Autodesk Fusion 360 part; units mm, degrees
(part 2 of 2)
sketch "Sketch5" plane through (0, 0, 0) normal (0, 0, -1) x (1, 0, 0)
  line L0 (-3.9005, -90.0072) -> (0, -96.4395)
  line L1 (0, -96.4395) -> (3.9005, -90.0072)
  arc A0 (-3.9005, -90.0072) -> (3.9005, -90.0072) centre (0, -96.4395) ccw
  line L2 (-4.2635, 5.5365) -> (-12.4173, 13.98)
  line L3 (-12.4173, 13.98) -> (-12.6168, 25.4085)
  line L4 (-12.6168, 25.4085) -> (-12.6168, 30.4597)
  line L5 (-12.6168, 30.4597) -> (-9.0451, 26.888)
  line L6 (-9.0451, 26.888) -> (-1.105, 18.6658)
  line L7 (-1.105, 18.6658) -> (-0.9001, 6.9296)
  line L8 (-0.9001, 6.9296) -> (-0.9137, 6.1554)
  line L9 (-0.9137, 6.1554) -> (-1.6405, 5.2892)
  line L10 (-1.6405, 5.2892) -> (-2.0296, 4.9)
  line L11 (-2.0296, 4.9) -> (-2.58, 4.9)
  line L12 (-2.58, 4.9) -> (-3.7064, 4.9985)
  line L13 (-3.7064, 4.9985) -> (-4.2635, 5.5365)
  line L14 (-28.1497, 7.7612) -> (-21.2885, 0.9)
  line L15 (-21.2885, 0.9) -> (-31.2992, 0.9)
  line L16 (-31.2992, 0.9) -> (-41.9773, 11.2116)
  line L17 (-41.9773, 11.2116) -> (-40.4166, 12.6168)
  line L18 (-40.4166, 12.6168) -> (-33.1778, 12.6168)
  line L19 (-33.1778, 12.6168) -> (-28.1497, 7.7612)
  line L20 (-21.2885, -0.9) -> (-28.1497, -7.7612)
  line L21 (-28.1497, -7.7612) -> (-33.1778, -12.6168)
  line L22 (-33.1778, -12.6168) -> (-40.4166, -12.6168)
  line L23 (-40.4166, -12.6168) -> (-41.9773, -11.2116)
  line L24 (-41.9773, -11.2116) -> (-31.2992, -0.9)
  line L25 (-31.2992, -0.9) -> (-21.2885, -0.9)
  line L26 (-33.8904, -0.9) -> (-43.3182, -10.0043)
  line L27 (-43.3182, -10.0043) -> (-53.4295, -0.9)
  line L28 (-53.4295, -0.9) -> (-33.8904, -0.9)
  line L29 (-93.238, 0) -> (-86.2449, 4.2406)
  line L30 (-86.2449, 4.2406) -> (-75.7491, 0)
  line L31 (-75.7491, 0) -> (-86.2449, -4.2406)
  line L32 (-86.2449, -4.2406) -> (-93.238, 0)
  line L33 (-53.4295, 0.9) -> (-43.3182, 10.0043)
  line L34 (-43.3182, 10.0043) -> (-33.8904, 0.9)
  line L35 (-33.8904, 0.9) -> (-53.4295, 0.9)
  line L36 (-18.6658, 1.105) -> (-26.888, 9.0451)
  line L37 (-26.888, 9.0451) -> (-30.4597, 12.6168)
  line L38 (-30.4597, 12.6168) -> (-25.4085, 12.6168)
  line L39 (-25.4085, 12.6168) -> (-13.98, 12.4173)
  line L40 (-13.98, 12.4173) -> (-5.5365, 4.2635)
  line L41 (-5.5365, 4.2635) -> (-4.9985, 3.7064)
  line L42 (-4.9985, 3.7064) -> (-4.9, 2.58)
  line L43 (-4.9, 2.58) -> (-4.9, 2.0296)
  line L44 (-4.9, 2.0296) -> (-5.2892, 1.6405)
  line L45 (-5.2892, 1.6405) -> (-6.1554, 0.9137)
  line L46 (-6.1554, 0.9137) -> (-6.9296, 0.9001)
  line L47 (-6.9296, 0.9001) -> (-18.6658, 1.105)
  arc A1 (-6.182, -86.2449) -> (6.182, -86.2449) centre (0, -96.4395) ccw
  line L48 (6.182, -86.2449) -> (0.9, -73.1716)
  line L49 (0.9, -73.1716) -> (0.9, -66.6716)
  line L50 (0.9, -66.6716) -> (8.1008, -75.8883)
  arc A2 (8.1008, -75.8883) -> (9.5193, -74.7801) centre (8.8101, -75.3342) ccw
  line L51 (9.5193, -74.7801) -> (0.9, -63.7479)
  line L52 (0.9, -63.7479) -> (0.9, -56.6479)
  line L53 (0.9, -56.6479) -> (14.9397, -72.7987)
  arc A3 (14.9397, -72.7987) -> (16.2982, -71.6178) centre (15.6189, -72.2083) ccw
  line L54 (16.2982, -71.6178) -> (11.9485, -66.6141)
  line L55 (11.9485, -66.6141) -> (15.3003, -65.847)
  arc A4 (15.3003, -65.847) -> (14.8988, -64.0923) centre (15.0995, -64.9697) ccw
  line L56 (14.8988, -64.0923) -> (10.6097, -65.074)
  line L57 (10.6097, -65.074) -> (1.8798, -55.0314)
  line L58 (1.8798, -55.0314) -> (14.4168, -41.1076)
  line L59 (14.4168, -41.1076) -> (14.4168, -34.8053)
  line L60 (14.4168, -34.8053) -> (18.8732, -39.2617)
  line L61 (18.8732, -39.2617) -> (37.5839, -40.2423)
  line L62 (37.5839, -40.2423) -> (38.5121, -53.5164)
  line L63 (38.5121, -53.5164) -> (34.7851, -55.8551)
  arc A5 (34.7851, -55.8551) -> (35.7419, -57.3798) centre (35.2635, -56.6175) ccw
  line L64 (35.7419, -57.3798) -> (38.6544, -55.5521)
  line L65 (38.6544, -55.5521) -> (39.1169, -62.166)
  arc A6 (39.1169, -62.166) -> (40.9125, -62.0404) centre (40.0147, -62.1032) ccw
  line L66 (40.9125, -62.0404) -> (39.4198, -40.6925)
  line L67 (39.4198, -40.6925) -> (44.4402, -45.713)
  line L68 (44.4402, -45.713) -> (46.1464, -59.6086)
  arc A7 (46.1464, -59.6086) -> (47.933, -59.3893) centre (47.0397, -59.499) ccw
  line L69 (47.933, -59.3893) -> (46.5076, -47.7804)
  line L70 (46.5076, -47.7804) -> (51.1038, -52.3766)
  line L71 (51.1038, -52.3766) -> (56.6131, -65.3557)
  line L72 (56.6131, -65.3557) -> (68.193, -68.193)
  line L73 (68.193, -68.193) -> (65.3557, -56.6131)
  line L74 (65.3557, -56.6131) -> (52.3766, -51.1038)
  line L75 (52.3766, -51.1038) -> (47.7804, -46.5076)
  line L76 (47.7804, -46.5076) -> (59.3893, -47.933)
  arc A8 (59.3893, -47.933) -> (59.6086, -46.1464) centre (59.499, -47.0397) ccw
  line L77 (59.6086, -46.1464) -> (45.713, -44.4402)
  line L78 (45.713, -44.4402) -> (40.6925, -39.4198)
  line L79 (40.6925, -39.4198) -> (62.0404, -40.9125)
  arc A9 (62.0404, -40.9125) -> (62.166, -39.1169) centre (62.1032, -40.0147) ccw
  line L80 (62.166, -39.1169) -> (55.5521, -38.6544)
  line L81 (55.5521, -38.6544) -> (57.3798, -35.7419)
  arc A10 (57.3798, -35.7419) -> (55.8551, -34.7851) centre (56.6175, -35.2635) ccw
  line L82 (55.8551, -34.7851) -> (53.5164, -38.5121)
  line L83 (53.5164, -38.5121) -> (40.2423, -37.5839)
  line L84 (40.2423, -37.5839) -> (39.2617, -18.8732)
  line L85 (39.2617, -18.8732) -> (34.8053, -14.4168)
  line L86 (34.8053, -14.4168) -> (41.1076, -14.4168)
  line L87 (41.1076, -14.4168) -> (55.0314, -1.8798)
  line L88 (55.0314, -1.8798) -> (65.074, -10.6097)
  line L89 (65.074, -10.6097) -> (64.0923, -14.8988)
  arc A11 (64.0923, -14.8988) -> (65.847, -15.3003) centre (64.9697, -15.0995) ccw
  line L90 (65.847, -15.3003) -> (66.6141, -11.9485)
  line L91 (66.6141, -11.9485) -> (71.6178, -16.2982)
  arc A12 (71.6178, -16.2982) -> (72.7987, -14.9397) centre (72.2083, -15.6189) ccw
  line L92 (72.7987, -14.9397) -> (56.6479, -0.9)
  line L93 (56.6479, -0.9) -> (63.7479, -0.9)
  line L94 (63.7479, -0.9) -> (74.7801, -9.5193)
  arc A13 (74.7801, -9.5193) -> (75.8883, -8.1008) centre (75.3342, -8.8101) ccw
  line L95 (75.8883, -8.1008) -> (66.6716, -0.9)
  line L96 (66.6716, -0.9) -> (73.1716, -0.9)
  line L97 (73.1716, -0.9) -> (86.2449, -6.182)
  line L98 (86.2449, -6.182) -> (96.4395, 0)
  line L99 (96.4395, 0) -> (86.2449, 6.182)
  line L100 (86.2449, 6.182) -> (73.1716, 0.9)
  line L101 (73.1716, 0.9) -> (66.6716, 0.9)
  line L102 (66.6716, 0.9) -> (75.8883, 8.1008)
  arc A14 (75.8883, 8.1008) -> (74.7801, 9.5193) centre (75.3342, 8.8101) ccw
  line L103 (74.7801, 9.5193) -> (63.7479, 0.9)
  line L104 (63.7479, 0.9) -> (56.6479, 0.9)
  line L105 (56.6479, 0.9) -> (72.7987, 14.9397)
  arc A15 (72.7987, 14.9397) -> (71.6178, 16.2982) centre (72.2083, 15.6189) ccw
  line L106 (71.6178, 16.2982) -> (66.6141, 11.9485)
  line L107 (66.6141, 11.9485) -> (65.847, 15.3003)
  arc A16 (65.847, 15.3003) -> (64.0923, 14.8988) centre (64.9697, 15.0995) ccw
  line L108 (64.0923, 14.8988) -> (65.074, 10.6097)
  line L109 (65.074, 10.6097) -> (55.0314, 1.8798)
  line L110 (55.0314, 1.8798) -> (41.1076, 14.4168)
  line L111 (41.1076, 14.4168) -> (34.8053, 14.4168)
  line L112 (34.8053, 14.4168) -> (39.2617, 18.8732)
  line L113 (39.2617, 18.8732) -> (40.2423, 37.5839)
  line L114 (40.2423, 37.5839) -> (53.5164, 38.5121)
  line L115 (53.5164, 38.5121) -> (55.8551, 34.7851)
  arc A17 (55.8551, 34.7851) -> (57.3798, 35.7419) centre (56.6175, 35.2635) ccw
  line L116 (57.3798, 35.7419) -> (55.5521, 38.6544)
  line L117 (55.5521, 38.6544) -> (62.166, 39.1169)
  arc A18 (62.166, 39.1169) -> (62.0404, 40.9125) centre (62.1032, 40.0147) ccw
  line L118 (62.0404, 40.9125) -> (40.6925, 39.4198)
  line L119 (40.6925, 39.4198) -> (45.713, 44.4402)
  line L120 (45.713, 44.4402) -> (59.6086, 46.1464)
  arc A19 (59.6086, 46.1464) -> (59.3893, 47.933) centre (59.499, 47.0397) ccw
  line L121 (59.3893, 47.933) -> (47.7804, 46.5076)
  line L122 (47.7804, 46.5076) -> (52.3766, 51.1038)
  line L123 (52.3766, 51.1038) -> (65.3557, 56.6131)
  line L124 (65.3557, 56.6131) -> (68.193, 68.193)
  line L125 (68.193, 68.193) -> (56.6131, 65.3557)
  line L126 (56.6131, 65.3557) -> (51.1038, 52.3766)
  line L127 (51.1038, 52.3766) -> (46.5076, 47.7804)
  line L128 (46.5076, 47.7804) -> (47.933, 59.3893)
  arc A20 (47.933, 59.3893) -> (46.1464, 59.6086) centre (47.0397, 59.499) ccw
  line L129 (46.1464, 59.6086) -> (44.4402, 45.713)
  line L130 (44.4402, 45.713) -> (39.4198, 40.6925)
  line L131 (39.4198, 40.6925) -> (40.9125, 62.0404)
  arc A21 (40.9125, 62.0404) -> (39.1169, 62.166) centre (40.0147, 62.1032) ccw
  line L132 (39.1169, 62.166) -> (38.6544, 55.5521)
  line L133 (38.6544, 55.5521) -> (35.7419, 57.3798)
  arc A22 (35.7419, 57.3798) -> (34.7851, 55.8551) centre (35.2635, 56.6175) ccw
  line L134 (34.7851, 55.8551) -> (38.5121, 53.5164)
  line L135 (38.5121, 53.5164) -> (37.5839, 40.2423)
  line L136 (37.5839, 40.2423) -> (18.8732, 39.2617)
  line L137 (18.8732, 39.2617) -> (14.4168, 34.8053)
  line L138 (14.4168, 34.8053) -> (14.4168, 41.1076)
  line L139 (14.4168, 41.1076) -> (1.8798, 55.0314)
  line L140 (1.8798, 55.0314) -> (10.6097, 65.074)
  line L141 (10.6097, 65.074) -> (14.8988, 64.0923)
  arc A23 (14.8988, 64.0923) -> (15.3003, 65.847) centre (15.0995, 64.9697) ccw
  line L142 (15.3003, 65.847) -> (11.9485, 66.6141)
  line L143 (11.9485, 66.6141) -> (16.2982, 71.6178)
  arc A24 (16.2982, 71.6178) -> (14.9397, 72.7987) centre (15.6189, 72.2083) ccw
  line L144 (14.9397, 72.7987) -> (0.9, 56.6479)
  line L145 (0.9, 56.6479) -> (0.9, 63.7479)
  line L146 (0.9, 63.7479) -> (9.5193, 74.7801)
  arc A25 (9.5193, 74.7801) -> (8.1008, 75.8883) centre (8.8101, 75.3342) ccw
  line L147 (8.1008, 75.8883) -> (0.9, 66.6716)
  line L148 (0.9, 66.6716) -> (0.9, 73.1716)
  line L149 (0.9, 73.1716) -> (6.182, 86.2449)
  line L150 (6.182, 86.2449) -> (0, 96.4395)
  line L151 (0, 96.4395) -> (-6.182, 86.2449)
  line L152 (-6.182, 86.2449) -> (-0.9, 73.1716)
  line L153 (-0.9, 73.1716) -> (-0.9, 66.6716)
  line L154 (-0.9, 66.6716) -> (-8.1008, 75.8883)
  arc A26 (-8.1008, 75.8883) -> (-9.5193, 74.7801) centre (-8.8101, 75.3342) ccw
  line L155 (-9.5193, 74.7801) -> (-0.9, 63.7479)
  line L156 (-0.9, 63.7479) -> (-0.9, 56.6479)
  line L157 (-0.9, 56.6479) -> (-14.9397, 72.7987)
  arc A27 (-14.9397, 72.7987) -> (-16.2982, 71.6178) centre (-15.6189, 72.2083) ccw
  line L158 (-16.2982, 71.6178) -> (-11.9485, 66.6141)
  line L159 (-11.9485, 66.6141) -> (-15.3003, 65.847)
  arc A28 (-15.3003, 65.847) -> (-14.8988, 64.0923) centre (-15.0995, 64.9697) ccw
  line L160 (-14.8988, 64.0923) -> (-10.6097, 65.074)
  line L161 (-10.6097, 65.074) -> (-1.8798, 55.0314)
  line L162 (-1.8798, 55.0314) -> (-14.4168, 41.1076)
  line L163 (-14.4168, 41.1076) -> (-14.4168, 34.8053)
  line L164 (-14.4168, 34.8053) -> (-18.8732, 39.2617)
  line L165 (-18.8732, 39.2617) -> (-37.5839, 40.2423)
  line L166 (-37.5839, 40.2423) -> (-38.5121, 53.5164)
  line L167 (-38.5121, 53.5164) -> (-34.7851, 55.8551)
  arc A29 (-34.7851, 55.8551) -> (-35.7419, 57.3798) centre (-35.2635, 56.6175) ccw
  line L168 (-35.7419, 57.3798) -> (-38.6544, 55.5521)
  line L169 (-38.6544, 55.5521) -> (-39.1169, 62.166)
  arc A30 (-39.1169, 62.166) -> (-40.9125, 62.0404) centre (-40.0147, 62.1032) ccw
  line L170 (-40.9125, 62.0404) -> (-39.4198, 40.6925)
  line L171 (-39.4198, 40.6925) -> (-44.4402, 45.713)
  line L172 (-44.4402, 45.713) -> (-46.1464, 59.6086)
  arc A31 (-46.1464, 59.6086) -> (-47.933, 59.3893) centre (-47.0397, 59.499) ccw
  line L173 (-47.933, 59.3893) -> (-46.5076, 47.7804)
  line L174 (-46.5076, 47.7804) -> (-51.1038, 52.3766)
  line L175 (-51.1038, 52.3766) -> (-56.6131, 65.3557)
  line L176 (-56.6131, 65.3557) -> (-68.193, 68.193)
  line L177 (-68.193, 68.193) -> (-65.3557, 56.6131)
  line L178 (-65.3557, 56.6131) -> (-52.3766, 51.1038)
  line L179 (-52.3766, 51.1038) -> (-47.7804, 46.5076)
  line L180 (-47.7804, 46.5076) -> (-59.3893, 47.933)
  arc A32 (-59.3893, 47.933) -> (-59.6086, 46.1464) centre (-59.499, 47.0397) ccw
  line L181 (-59.6086, 46.1464) -> (-45.713, 44.4402)
  line L182 (-45.713, 44.4402) -> (-40.6925, 39.4198)
  line L183 (-40.6925, 39.4198) -> (-62.0404, 40.9125)
  arc A33 (-62.0404, 40.9125) -> (-62.166, 39.1169) centre (-62.1032, 40.0147) ccw
  line L184 (-62.166, 39.1169) -> (-55.5521, 38.6544)
  line L185 (-55.5521, 38.6544) -> (-57.3798, 35.7419)
  arc A34 (-57.3798, 35.7419) -> (-55.8551, 34.7851) centre (-56.6175, 35.2635) ccw
  line L186 (-55.8551, 34.7851) -> (-53.5164, 38.5121)
  line L187 (-53.5164, 38.5121) -> (-40.2423, 37.5839)
  line L188 (-40.2423, 37.5839) -> (-39.2617, 18.8732)
  line L189 (-39.2617, 18.8732) -> (-34.8053, 14.4168)
  line L190 (-34.8053, 14.4168) -> (-41.1076, 14.4168)
  line L191 (-41.1076, 14.4168) -> (-55.0314, 1.8798)
  line L192 (-55.0314, 1.8798) -> (-65.074, 10.6097)
  line L193 (-65.074, 10.6097) -> (-64.0923, 14.8988)
  arc A35 (-64.0923, 14.8988) -> (-65.847, 15.3003) centre (-64.9697, 15.0995) ccw
  line L194 (-65.847, 15.3003) -> (-66.6141, 11.9485)
  line L195 (-66.6141, 11.9485) -> (-71.6178, 16.2982)
  arc A36 (-71.6178, 16.2982) -> (-72.7987, 14.9397) centre (-72.2083, 15.6189) ccw
  line L196 (-72.7987, 14.9397) -> (-56.6479, 0.9)
  line L197 (-56.6479, 0.9) -> (-63.7479, 0.9)
  line L198 (-63.7479, 0.9) -> (-74.7801, 9.5193)
  arc A37 (-74.7801, 9.5193) -> (-75.8883, 8.1008) centre (-75.3342, 8.8101) ccw
  line L199 (-75.8883, 8.1008) -> (-66.6716, 0.9)
  line L200 (-66.6716, 0.9) -> (-73.1716, 0.9)
  line L201 (-73.1716, 0.9) -> (-86.2449, 6.182)
  line L202 (-86.2449, 6.182) -> (-96.4395, 0)
  line L203 (-96.4395, 0) -> (-86.2449, -6.182)
  line L204 (-86.2449, -6.182) -> (-73.1716, -0.9)
  line L205 (-73.1716, -0.9) -> (-66.6716, -0.9)
  line L206 (-66.6716, -0.9) -> (-75.8883, -8.1008)
  arc A38 (-75.8883, -8.1008) -> (-74.7801, -9.5193) centre (-75.3342, -8.8101) ccw
  line L207 (-74.7801, -9.5193) -> (-63.7479, -0.9)
  line L208 (-63.7479, -0.9) -> (-56.6479, -0.9)
  line L209 (-56.6479, -0.9) -> (-72.7987, -14.9397)
  arc A39 (-72.7987, -14.9397) -> (-71.6178, -16.2982) centre (-72.2083, -15.6189) ccw
  line L210 (-71.6178, -16.2982) -> (-66.6141, -11.9485)
  line L211 (-66.6141, -11.9485) -> (-65.847, -15.3003)
  arc A40 (-65.847, -15.3003) -> (-64.0923, -14.8988) centre (-64.9697, -15.0995) ccw
  line L212 (-64.0923, -14.8988) -> (-65.074, -10.6097)
  line L213 (-65.074, -10.6097) -> (-55.0314, -1.8798)
  line L214 (-55.0314, -1.8798) -> (-41.1076, -14.4168)
  line L215 (-41.1076, -14.4168) -> (-34.8053, -14.4168)
  line L216 (-34.8053, -14.4168) -> (-39.2617, -18.8732)
  line L217 (-39.2617, -18.8732) -> (-40.2423, -37.5839)
  line L218 (-40.2423, -37.5839) -> (-53.5164, -38.5121)
  line L219 (-53.5164, -38.5121) -> (-55.8551, -34.7851)
  arc A41 (-55.8551, -34.7851) -> (-57.3798, -35.7419) centre (-56.6175, -35.2635) ccw
  line L220 (-57.3798, -35.7419) -> (-55.5521, -38.6544)
  line L221 (-55.5521, -38.6544) -> (-62.166, -39.1169)
  arc A42 (-62.166, -39.1169) -> (-62.0404, -40.9125) centre (-62.1032, -40.0147) ccw
  line L222 (-62.0404, -40.9125) -> (-40.6925, -39.4198)
  line L223 (-40.6925, -39.4198) -> (-45.713, -44.4402)
  line L224 (-45.713, -44.4402) -> (-59.6086, -46.1464)
  arc A43 (-59.6086, -46.1464) -> (-59.3893, -47.933) centre (-59.499, -47.0397) ccw
  line L225 (-59.3893, -47.933) -> (-47.7804, -46.5076)
  line L226 (-47.7804, -46.5076) -> (-52.3766, -51.1038)
  line L227 (-52.3766, -51.1038) -> (-65.3557, -56.6131)
  line L228 (-65.3557, -56.6131) -> (-68.193, -68.193)
  line L229 (-68.193, -68.193) -> (-56.6131, -65.3557)
  line L230 (-56.6131, -65.3557) -> (-51.1038, -52.3766)
  line L231 (-51.1038, -52.3766) -> (-46.5076, -47.7804)
  line L232 (-46.5076, -47.7804) -> (-47.933, -59.3893)
  arc A44 (-47.933, -59.3893) -> (-46.1464, -59.6086) centre (-47.0397, -59.499) ccw
  line L233 (-46.1464, -59.6086) -> (-44.4402, -45.713)
  line L234 (-44.4402, -45.713) -> (-39.4198, -40.6925)
  line L235 (-39.4198, -40.6925) -> (-40.9125, -62.0404)
  arc A45 (-40.9125, -62.0404) -> (-39.1169, -62.166) centre (-40.0147, -62.1032) ccw
  line L236 (-39.1169, -62.166) -> (-38.6544, -55.5521)
  line L237 (-38.6544, -55.5521) -> (-35.7419, -57.3798)
  arc A46 (-35.7419, -57.3798) -> (-34.7851, -55.8551) centre (-35.2635, -56.6175) ccw
  line L238 (-34.7851, -55.8551) -> (-38.5121, -53.5164)
  line L239 (-38.5121, -53.5164) -> (-37.5839, -40.2423)
  line L240 (-37.5839, -40.2423) -> (-18.8732, -39.2617)
  line L241 (-18.8732, -39.2617) -> (-14.4168, -34.8053)
  line L242 (-14.4168, -34.8053) -> (-14.4168, -41.1076)
  line L243 (-14.4168, -41.1076) -> (-1.8798, -55.0314)
  line L244 (-1.8798, -55.0314) -> (-10.6097, -65.074)
  line L245 (-10.6097, -65.074) -> (-14.8988, -64.0923)
  arc A47 (-14.8988, -64.0923) -> (-15.3003, -65.847) centre (-15.0995, -64.9697) ccw
  line L246 (-15.3003, -65.847) -> (-11.9485, -66.6141)
  line L247 (-11.9485, -66.6141) -> (-16.2982, -71.6178)
  arc A48 (-16.2982, -71.6178) -> (-14.9397, -72.7987) centre (-15.6189, -72.2083) ccw
  line L248 (-14.9397, -72.7987) -> (-0.9, -56.6479)
  line L249 (-0.9, -56.6479) -> (-0.9, -63.7479)
  line L250 (-0.9, -63.7479) -> (-9.5193, -74.7801)
  arc A49 (-9.5193, -74.7801) -> (-8.1008, -75.8883) centre (-8.8101, -75.3342) ccw
  line L251 (-8.1008, -75.8883) -> (-0.9, -66.6716)
  line L252 (-0.9, -66.6716) -> (-0.9, -73.1716)
  line L253 (-0.9, -73.1716) -> (-6.182, -86.2449)
  line L254 (4.9, -2.0296) -> (5.2892, -1.6405)
  line L255 (5.2892, -1.6405) -> (6.1554, -0.9137)
  line L256 (6.1554, -0.9137) -> (6.9296, -0.9001)
  line L257 (6.9296, -0.9001) -> (18.6658, -1.105)
  line L258 (18.6658, -1.105) -> (26.888, -9.0451)
  line L259 (26.888, -9.0451) -> (30.4597, -12.6168)
  line L260 (30.4597, -12.6168) -> (25.4085, -12.6168)
  line L261 (25.4085, -12.6168) -> (13.98, -12.4173)
  line L262 (13.98, -12.4173) -> (5.5365, -4.2635)
  line L263 (5.5365, -4.2635) -> (4.9985, -3.7064)
  line L264 (4.9985, -3.7064) -> (4.9, -2.58)
  line L265 (4.9, -2.58) -> (4.9, -2.0296)
  line L266 (-25.3928, -14.4168) -> (-15.6896, -14.4168)
  line L267 (-15.6896, -14.4168) -> (-22.7683, -21.4955)
  line L268 (-22.7683, -21.4955) -> (-37.6102, -21.7546)
  line L269 (-37.6102, -21.7546) -> (-37.5003, -19.6574)
  line L270 (-37.5003, -19.6574) -> (-32.3817, -14.5388)
  line L271 (-32.3817, -14.5388) -> (-25.3928, -14.4168)
  line L272 (-14.4168, 15.6896) -> (-21.4955, 22.7683)
  line L273 (-21.4955, 22.7683) -> (-21.7546, 37.6102)
  line L274 (-21.7546, 37.6102) -> (-19.6574, 37.5003)
  line L275 (-19.6574, 37.5003) -> (-14.5388, 32.3817)
  line L276 (-14.5388, 32.3817) -> (-14.4168, 25.3928)
  line L277 (-14.4168, 25.3928) -> (-14.4168, 15.6896)
  line L278 (28.1497, 7.7612) -> (33.1778, 12.6168)
  line L279 (33.1778, 12.6168) -> (40.4166, 12.6168)
  line L280 (40.4166, 12.6168) -> (41.9773, 11.2116)
  line L281 (41.9773, 11.2116) -> (31.2992, 0.9)
  line L282 (31.2992, 0.9) -> (21.2885, 0.9)
  line L283 (21.2885, 0.9) -> (28.1497, 7.7612)
  line L284 (14.4168, -25.3928) -> (14.4168, -15.6896)
  line L285 (14.4168, -15.6896) -> (21.4955, -22.7683)
  line L286 (21.4955, -22.7683) -> (21.7546, -37.6102)
  line L287 (21.7546, -37.6102) -> (19.6574, -37.5003)
  line L288 (19.6574, -37.5003) -> (14.5388, -32.3817)
  line L289 (14.5388, -32.3817) -> (14.4168, -25.3928)
  line L290 (15.6896, -14.4168) -> (25.3928, -14.4168)
  line L291 (25.3928, -14.4168) -> (32.3817, -14.5388)
  line L292 (32.3817, -14.5388) -> (37.5003, -19.6574)
  line L293 (37.5003, -19.6574) -> (37.6102, -21.7546)
  line L294 (37.6102, -21.7546) -> (22.7683, -21.4955)
  line L295 (22.7683, -21.4955) -> (15.6896, -14.4168)
  line L296 (24.6006, -23.3278) -> (37.7047, -23.5565)
  line L297 (37.7047, -23.5565) -> (38.4168, -37.144)
  line L298 (38.4168, -37.144) -> (24.6006, -23.3278)
  line L299 (65.9292, -65.9292) -> (57.9858, -63.9829)
  line L300 (57.9858, -63.9829) -> (53.5627, -53.5627)
  line L301 (53.5627, -53.5627) -> (63.9829, -57.9858)
  line L302 (63.9829, -57.9858) -> (65.9292, -65.9292)
  line L303 (37.144, -38.4168) -> (23.5565, -37.7047)
  line L304 (23.5565, -37.7047) -> (23.3278, -24.6006)
  line L305 (23.3278, -24.6006) -> (37.144, -38.4168)
  line L306 (7.7612, -28.1497) -> (12.6168, -33.1778)
  line L307 (12.6168, -33.1778) -> (12.6168, -40.4166)
  line L308 (12.6168, -40.4166) -> (11.2116, -41.9773)
  line L309 (11.2116, -41.9773) -> (0.9, -31.2992)
  line L310 (0.9, -31.2992) -> (0.9, -21.2885)
  line L311 (0.9, -21.2885) -> (7.7612, -28.1497)
  line L312 (0.9, -33.8904) -> (10.0043, -43.3182)
  line L313 (10.0043, -43.3182) -> (0.9, -53.4295)
  line L314 (0.9, -53.4295) -> (0.9, -33.8904)
  line L315 (0, -93.238) -> (-4.2406, -86.2449)
  line L316 (-4.2406, -86.2449) -> (0, -75.7491)
  line L317 (0, -75.7491) -> (4.2406, -86.2449)
  line L318 (4.2406, -86.2449) -> (0, -93.238)
  line L319 (-0.9, -53.4295) -> (-10.0043, -43.3182)
  line L320 (-10.0043, -43.3182) -> (-0.9, -33.8904)
  line L321 (-0.9, -33.8904) -> (-0.9, -53.4295)
  line L322 (-7.7612, -28.1497) -> (-0.9, -21.2885)
  line L323 (-0.9, -21.2885) -> (-0.9, -31.2992)
  line L324 (-0.9, -31.2992) -> (-11.2116, -41.9773)
  line L325 (-11.2116, -41.9773) -> (-12.6168, -40.4166)
  line L326 (-12.6168, -40.4166) -> (-12.6168, -33.1778)
  line L327 (-12.6168, -33.1778) -> (-7.7612, -28.1497)
  line L328 (-23.3278, -24.6006) -> (-23.5565, -37.7047)
  line L329 (-23.5565, -37.7047) -> (-37.144, -38.4168)
  line L330 (-37.144, -38.4168) -> (-23.3278, -24.6006)
  line L331 (-65.9292, -65.9292) -> (-63.9829, -57.9858)
  line L332 (-63.9829, -57.9858) -> (-53.5627, -53.5627)
  line L333 (-53.5627, -53.5627) -> (-57.9858, -63.9829)
  line L334 (-57.9858, -63.9829) -> (-65.9292, -65.9292)
  line L335 (-38.4168, -37.144) -> (-37.7047, -23.5565)
  line L336 (-37.7047, -23.5565) -> (-24.6006, -23.3278)
  line L337 (-24.6006, -23.3278) -> (-38.4168, -37.144)
  line L338 (-14.4168, -25.3928) -> (-14.5388, -32.3817)
  line L339 (-14.5388, -32.3817) -> (-19.6574, -37.5003)
  line L340 (-19.6574, -37.5003) -> (-21.7546, -37.6102)
  line L341 (-21.7546, -37.6102) -> (-21.4955, -22.7683)
  line L342 (-21.4955, -22.7683) -> (-14.4168, -15.6896)
  line L343 (-14.4168, -15.6896) -> (-14.4168, -25.3928)
  line L344 (53.4295, -0.9) -> (43.3182, -10.0043)
  line L345 (43.3182, -10.0043) -> (33.8904, -0.9)
  line L346 (33.8904, -0.9) -> (53.4295, -0.9)
  line L347 (93.238, 0) -> (86.2449, -4.2406)
  line L348 (86.2449, -4.2406) -> (75.7491, 0)
  line L349 (75.7491, 0) -> (86.2449, 4.2406)
  line L350 (86.2449, 4.2406) -> (93.238, 0)
  line L351 (33.8904, 0.9) -> (43.3182, 10.0043)
  line L352 (43.3182, 10.0043) -> (53.4295, 0.9)
  line L353 (53.4295, 0.9) -> (33.8904, 0.9)
  line L354 (28.1497, -7.7612) -> (21.2885, -0.9)
  line L355 (21.2885, -0.9) -> (31.2992, -0.9)
  line L356 (31.2992, -0.9) -> (41.9773, -11.2116)
  line L357 (41.9773, -11.2116) -> (40.4166, -12.6168)
  line L358 (40.4166, -12.6168) -> (33.1778, -12.6168)
  line L359 (33.1778, -12.6168) -> (28.1497, -7.7612)
  line L360 (23.3278, 24.6006) -> (23.5565, 37.7047)
  line L361 (23.5565, 37.7047) -> (37.144, 38.4168)
  line L362 (37.144, 38.4168) -> (23.3278, 24.6006)
  line L363 (65.9292, 65.9292) -> (63.9829, 57.9858)
  line L364 (63.9829, 57.9858) -> (53.5627, 53.5627)
  line L365 (53.5627, 53.5627) -> (57.9858, 63.9829)
  line L366 (57.9858, 63.9829) -> (65.9292, 65.9292)
  line L367 (38.4168, 37.144) -> (37.7047, 23.5565)
  line L368 (37.7047, 23.5565) -> (24.6006, 23.3278)
  line L369 (24.6006, 23.3278) -> (38.4168, 37.144)
  line L370 (15.6896, 14.4168) -> (22.7683, 21.4955)
  line L371 (22.7683, 21.4955) -> (37.6102, 21.7546)
  line L372 (37.6102, 21.7546) -> (37.5003, 19.6574)
  line L373 (37.5003, 19.6574) -> (32.3817, 14.5388)
  line L374 (32.3817, 14.5388) -> (25.3928, 14.4168)
  line L375 (25.3928, 14.4168) -> (15.6896, 14.4168)
  line L376 (14.4168, 25.3928) -> (14.5388, 32.3817)
  line L377 (14.5388, 32.3817) -> (19.6574, 37.5003)
  line L378 (19.6574, 37.5003) -> (21.7546, 37.6102)
  line L379 (21.7546, 37.6102) -> (21.4955, 22.7683)
  line L380 (21.4955, 22.7683) -> (14.4168, 15.6896)
  line L381 (14.4168, 15.6896) -> (14.4168, 25.3928)
  line L382 (0.9, 21.2885) -> (0.9, 31.2992)
  line L383 (0.9, 31.2992) -> (11.2116, 41.9773)
  line L384 (11.2116, 41.9773) -> (12.6168, 40.4166)
  line L385 (12.6168, 40.4166) -> (12.6168, 33.1778)
  line L386 (12.6168, 33.1778) -> (7.7612, 28.1497)
  line L387 (7.7612, 28.1497) -> (0.9, 21.2885)
  line L388 (-0.9, 33.8904) -> (-10.0043, 43.3182)
  line L389 (-10.0043, 43.3182) -> (-0.9, 53.4295)
  line L390 (-0.9, 53.4295) -> (-0.9, 33.8904)
  line L391 (0, 93.238) -> (4.2406, 86.2449)
  line L392 (4.2406, 86.2449) -> (0, 75.7491)
  line L393 (0, 75.7491) -> (-4.2406, 86.2449)
  line L394 (-4.2406, 86.2449) -> (0, 93.238)
  line L395 (0.9, 53.4295) -> (10.0043, 43.3182)
  line L396 (10.0043, 43.3182) -> (0.9, 33.8904)
  line L397 (0.9, 33.8904) -> (0.9, 53.4295)
  line L398 (-7.7612, 28.1497) -> (-12.6168, 33.1778)
  line L399 (-12.6168, 33.1778) -> (-12.6168, 40.4166)
  line L400 (-12.6168, 40.4166) -> (-11.2116, 41.9773)
  line L401 (-11.2116, 41.9773) -> (-0.9, 31.2992)
  line L402 (-0.9, 31.2992) -> (-0.9, 21.2885)
  line L403 (-0.9, 21.2885) -> (-7.7612, 28.1497)
  line L404 (-37.144, 38.4168) -> (-23.5565, 37.7047)
  line L405 (-23.5565, 37.7047) -> (-23.3278, 24.6006)
  line L406 (-23.3278, 24.6006) -> (-37.144, 38.4168)
  line L407 (-65.9292, 65.9292) -> (-57.9858, 63.9829)
  line L408 (-57.9858, 63.9829) -> (-53.5627, 53.5627)
  line L409 (-53.5627, 53.5627) -> (-63.9829, 57.9858)
  line L410 (-63.9829, 57.9858) -> (-65.9292, 65.9292)
  line L411 (-24.6006, 23.3278) -> (-37.7047, 23.5565)
  line L412 (-37.7047, 23.5565) -> (-38.4168, 37.144)
  line L413 (-38.4168, 37.144) -> (-24.6006, 23.3278)
  line L414 (-2.0296, -4.9) -> (-1.6405, -5.2892)
  line L415 (-1.6405, -5.2892) -> (-0.9137, -6.1554)
  line L416 (-0.9137, -6.1554) -> (-0.9001, -6.9296)
  line L417 (-0.9001, -6.9296) -> (-1.105, -18.6658)
  line L418 (-1.105, -18.6658) -> (-9.0451, -26.888)
  line L419 (-9.0451, -26.888) -> (-12.6168, -30.4597)
  line L420 (-12.6168, -30.4597) -> (-12.6168, -25.4085)
  line L421 (-12.6168, -25.4085) -> (-12.4173, -13.98)
  line L422 (-12.4173, -13.98) -> (-4.2635, -5.5365)
  line L423 (-4.2635, -5.5365) -> (-3.7064, -4.9985)
  line L424 (-3.7064, -4.9985) -> (-2.58, -4.9)
  line L425 (-2.58, -4.9) -> (-2.0296, -4.9)
  line L426 (2.58, -4.9) -> (3.7064, -4.9985)
  line L427 (3.7064, -4.9985) -> (4.2635, -5.5365)
  line L428 (4.2635, -5.5365) -> (12.4173, -13.98)
  line L429 (12.4173, -13.98) -> (12.6168, -25.4085)
  line L430 (12.6168, -25.4085) -> (12.6168, -30.4597)
  line L431 (12.6168, -30.4597) -> (9.0451, -26.888)
  line L432 (9.0451, -26.888) -> (1.105, -18.6658)
  line L433 (1.105, -18.6658) -> (0.9001, -6.9296)
  line L434 (0.9001, -6.9296) -> (0.9137, -6.1554)
  line L435 (0.9137, -6.1554) -> (1.6405, -5.2892)
  line L436 (1.6405, -5.2892) -> (2.0296, -4.9)
  line L437 (2.0296, -4.9) -> (2.58, -4.9)
  line L438 (4.9, 2.58) -> (4.9985, 3.7064)
  line L439 (4.9985, 3.7064) -> (5.5365, 4.2635)
  line L440 (5.5365, 4.2635) -> (13.98, 12.4173)
  line L441 (13.98, 12.4173) -> (25.4085, 12.6168)
  line L442 (25.4085, 12.6168) -> (30.4597, 12.6168)
  line L443 (30.4597, 12.6168) -> (26.888, 9.0451)
  line L444 (26.888, 9.0451) -> (18.6658, 1.105)
  line L445 (18.6658, 1.105) -> (6.9296, 0.9001)
  line L446 (6.9296, 0.9001) -> (6.1554, 0.9137)
  line L447 (6.1554, 0.9137) -> (5.2892, 1.6405)
  line L448 (5.2892, 1.6405) -> (4.9, 2.0296)
  line L449 (4.9, 2.0296) -> (4.9, 2.58)
  line L450 (2.0296, 4.9) -> (1.6405, 5.2892)
  line L451 (1.6405, 5.2892) -> (0.9137, 6.1554)
  line L452 (0.9137, 6.1554) -> (0.9001, 6.9296)
  line L453 (0.9001, 6.9296) -> (1.105, 18.6658)
  line L454 (1.105, 18.6658) -> (9.0451, 26.888)
  line L455 (9.0451, 26.888) -> (12.6168, 30.4597)
  line L456 (12.6168, 30.4597) -> (12.6168, 25.4085)
  line L457 (12.6168, 25.4085) -> (12.4173, 13.98)
  line L458 (12.4173, 13.98) -> (4.2635, 5.5365)
  line L459 (4.2635, 5.5365) -> (3.7064, 4.9985)
  line L460 (3.7064, 4.9985) -> (2.58, 4.9)
  line L461 (2.58, 4.9) -> (2.0296, 4.9)
  line L462 (-15.6896, 14.4168) -> (-25.3928, 14.4168)
  line L463 (-25.3928, 14.4168) -> (-32.3817, 14.5388)
  line L464 (-32.3817, 14.5388) -> (-37.5003, 19.6574)
  line L465 (-37.5003, 19.6574) -> (-37.6102, 21.7546)
  line L466 (-37.6102, 21.7546) -> (-22.7683, 21.4955)
  line L467 (-22.7683, 21.4955) -> (-15.6896, 14.4168)
  line L468 (-30.4597, -12.6168) -> (-26.888, -9.0451)
  line L469 (-26.888, -9.0451) -> (-18.6658, -1.105)
  line L470 (-18.6658, -1.105) -> (-6.9296, -0.9001)
  line L471 (-6.9296, -0.9001) -> (-6.1554, -0.9137)
  line L472 (-6.1554, -0.9137) -> (-5.2892, -1.6405)
  line L473 (-5.2892, -1.6405) -> (-4.9, -2.0296)
  line L474 (-4.9, -2.0296) -> (-4.9, -2.58)
  line L475 (-4.9, -2.58) -> (-4.9985, -3.7064)
  line L476 (-4.9985, -3.7064) -> (-5.5365, -4.2635)
  line L477 (-5.5365, -4.2635) -> (-13.98, -12.4173)
  line L478 (-13.98, -12.4173) -> (-25.4085, -12.6168)
  line L479 (-25.4085, -12.6168) -> (-30.4597, -12.6168)
extrude "Extrude5" add sketch "Sketch5" against normal up to surface (5 mm away) separate body contours L2 L3 L4 L5 L6 L7 L8 L9 L10 L11 L12 L13 | L14 L15 L16 L17 L18 L19 | L20 L21 L22 L23 L24 L25 | L26 L27 L28 | L29 L30 L31 L32 | L33 L34 L35 | L36 L37 L38 L39 L40 L41 L42 L43 L44 L45 L46 L47 | L254 L255 L256 L257 L258 L259 L260 L261 L262 L263 L264 L265 | L266 L267 L268 L269 L270 L271 | L272 L273 L274 L275 L276 L277 | L278 L279 L280 L281 L282 L283 | L284 L285 L286 L287 L288 L289 | L290 L291 L292 L293 L294 L295 | L296 L297 L298 | L299 L300 L301 L302 | L303 L304 L305 | L306 L307 L308 L309 L310 L311 | L312 L313 L314 | L315 L316 L317 L318 | L319 L320 L321 | L322 L323 L324 L325 L326 L327 | L328 L329 L330 | L331 L332 L333 L334 | L335 L336 L337 | L338 L339 L340 L341 L342 L343 | L344 L345 L346 | L347 L348 L349 L350 | L351 L352 L353 | L354 L355 L356 L357 L358 L359 | L360 L361 L362 | L363 L364 L365 L366 | L367 L368 L369 | L370 L371 L372 L373 L374 L375 | L376 L377 L378 L379 L380 L381 | L382 L383 L384 L385 L386 L387 | L388 L389 L390 | L391 L392 L393 L394 | L395 L396 L397 | L398 L399 L400 L401 L402 L403 | L404 L405 L406 | L407 L408 L409 L410 | L411 L412 L413 | L414 L415 L416 L417 L418 L419 L420 L421 L422 L423 L424 L425 | L426 L427 L428 L429 L430 L431 L432 L433 L434 L435 L436 L437 | L438 L439 L440 L441 L442 L443 L444 L445 L446 L447 L448 L449 | L450 L451 L452 L453 L454 L455 L456 L457 L458 L459 L460 L461 | L462 L463 L464 L465 L466 L467 | L468 L469 L470 L471 L472 L473 L474 L475 L476 L477 L478 L479 makes body 9 at (-58.5105, 58.5105, 0) makes body 10 at (0.9, 46.9165, 1.6667) makes body 11 at (-19.263, 30.9201, 0) makes body 12 at (-13.1918, 4.8075, 0) makes body 13 at (-35.4848, -8.2428, 0) makes body 14 at (-27.9332, -29.206, 1.6667) makes body 15 at (-8.2428, -35.4848, 0) makes body 16 at (58.5105, -58.5105, 0) makes body 17 at (29.206, -27.9332, 3.3333) makes body 18 at (13.1918, -4.8075, 0) makes body 19 at (27.9332, 29.206, 1.6667) makes body 20 at (4.8075, 13.1918, 0) makes body 21 at (19.263, 30.9201, 0) makes body 22 at (40.4035, 0.9, 1.6667) makes body 23 at (46.9165, -0.9, 1.6667) makes body 24 at (32.5386, -33.8114, 1.6667) makes body 25 at (8.2428, -35.4848, 0) makes body 26 at (-5.9286, -12.7274, 0) makes body 27 at (-33.8114, -32.5386, 3.3333) makes body 28 at (-40.4035, -0.9, 1.6667) makes body 29 at (-30.9201, 19.263, 0) makes body 30 at (-5.9286, 12.7274, 0) makes body 31 at (8.2428, 35.4848, 0) makes body 32 at (-82.7463, 0, 0) makes body 33 at (0, 82.7463, 0) makes body 34 at (-0.9, 40.4035, 1.6667) makes body 35 at (-32.5386, 33.8114, 3.3333) makes body 36 at (-35.4848, 8.2428, 0) makes body 37 at (-13.1918, -4.8075, 0) makes body 38 at (-19.263, -30.9201, 0) makes body 39 at (-0.9, -46.9165, 1.6667) makes body 40 at (5.9286, -12.7274, 0) makes body 41 at (30.9201, -19.263, 0) makes body 42 at (35.4848, -8.2428, 0) makes body 43 at (33.8114, 32.5386, 1.6667) makes body 44 at (13.1918, 4.8075, 0) makes body 45 at (30.9201, 19.263, 0) makes body 46 at (35.4848, 8.2428, 0) makes body 47 at (82.7463, 0, 0) makes body 48 at (19.263, -30.9201, 0) makes body 49 at (0.9, -40.4035, 1.6667) makes body 50 at (0, -82.7463, 0) makes body 51 at (-30.9201, -19.263, 0) makes body 52 at (-46.9165, 0.9, 1.6667) makes body 53 at (-29.206, 27.9332, 1.6667) makes body 54 at (-8.2428, 35.4848, 0) makes body 55 at (58.5105, 58.5105, 0) makes body 56 at (-58.5105, -58.5105, 0)
equation "d464 = 80 °"
equation "d466 = d463"
equation "d468 = 158 °"
equation "d475 = ( 1.8 / 2 ) * 1 mm"
equation "d476 = 142 °"
equation "d480 = d474"
equation "d482 = 139 °"
equation "d483 = d474"
equation "d493 = 45 °"
equation "d495 = d492"
equation "d496 = d492"
equation "d497 = d492"
equation "d498 = d492"
equation "d499 = 97 °"
equation "d500 = 136 °"
